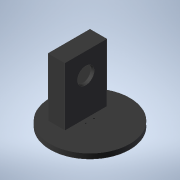
# Autodesk Inventor part: NBase top
Saved by Autodesk Inventor 2022 (Build 260153000, 153)
## iProperties
Created: 2022-02-11
Part Number: NBase top
Material: Generic
Document SubType Name: Modeling
Designer: Alexa
Density: 1 g/cm^3
Appearance: Default
Author: Alexa
Autodesk Inventor part; units mm, degrees
ref_plane "YZ Plane" through (0, 0, 0) normal (1, 0, 0) x (0, 1, 0)
ref_plane "XZ Plane" through (0, 0, 0) normal (0, 1, 0) x (-1, 0, 0)
ref_plane "XY Plane" through (0, 0, 0) normal (0, 0, 1) x (1, 0, 0)
sketch "Sketch1" plane through (0, 0, 0) normal (0, 1, 0) x (-1, 0, 0)
  circle A0 centre (0, 0) radius 47.5
  dimension "d0" = 95
  constraints: 1 centre point, 1 coincident
  measures "d0" diameter of A0
extrude "Extrusion1" add sketch "Sketch1" along normal blind 6
sketch "Sketch2" plane through (0, 6, 0) normal (0, 1, 0) x (1, 0, 0)
  circle A0 centre (0, 0) radius 10
  circle A1 centre (0, 5) radius 1
  circle A2 centre (0, -5) radius 1
  dimension "d3" = 20
  dimension "d4" = 2
  dimension "d5" = 2
  constraints: 3 centre point, 1 coincident
  measures "d3" diameter of A0
  measures "d4" diameter of A1
  measures "d5" diameter of A2
extrude "Extrusion2" cut sketch "Sketch2" against normal blind 23.4625 contours A1 | A2
sketch "Sketch3" plane through (0, 0, 0) normal (0, -1, 0) x (1, 0, 0)
  circle A0 centre (0, 0) radius 10
  constraints: 1 centre point, 1 coincident
sketch "Sketch4" plane through (0, 6, 0) normal (0, 1, 0) x (1, 0, 0)
  line L0 (0, 0) -> (-10, 0)
  line L1 (-10, 0) -> (-10, 25)
  line L2 (-10, 25) -> (0, 25)
  line L3 (0, 25) -> (0, 0)
  line L4 (0, 0) -> (-5, 0)
  line L5 (-5, 0) -> (-5, 25)
  line L6 (-5, 25) -> (0, 25)
  line L7 (0, 25) -> (0, 0)
  line L8 (-5, 25) -> (-20, 25)
  line L9 (-20, 25) -> (-20, -25)
  line L10 (-20, -25) -> (-5, -25)
  line L11 (-5, -25) -> (-5, 25)
  line L12 (-5, 25) -> (-25, 25)
  line L13 (-25, 25) -> (-25, -25)
  line L14 (-25, -25) -> (-5, -25)
  line L15 (-5, -25) -> (-5, 25)
  dimension "d9" = 10
  dimension "d10" = 25
  dimension "d11" = 15
  dimension "d12" = 50
  dimension "d13" = 20
  constraints: 32 end point, 8 parallel, 4 horizontal, 4 perpendicular, 1 midpoint
  measures "d9" distance of L1.end L2.end
  measures "d10" distance of L0.end L1.end
  measures "d11" distance of L10.end L9.end
  measures "d12" distance of L9.end L8.end
  measures "d13" distance of L14.end L13.end
extrude "Extrusion3" add sketch "Sketch4" along normal blind 70 contours L11 L10 L9 L8 L1 L0 | L0 L1 L2 L5 | L14 L13 L12 L9
sketch "Sketch5" plane through (-25, 6, -25) normal (-1, 0, 0) x (0, 0, 1)
  line L0 (0, 0) -> (0, 70) projected
  line L1 (50, 0) -> (50, 70) projected
  line L2 (0, 70) -> (50, 70)
  line L3 (50, 70) -> (50, 0)
  line L4 (50, 0) -> (0, 0)
  line L5 (0, 0) -> (0, 70)
  line L6 (50, 70) -> (0, 70) projected
  line L7 (72.5, 0) -> (-22.5, 0) projected
  line L8 (0, 70) -> (25, 70)
  line L9 (25, 70) -> (25, 0)
  line L10 (25, 0) -> (0, 0)
  line L11 (0, 0) -> (0, 70)
  line L12 (25, 35) -> (15, 35)
  line L13 (15, 35) -> (15, 15)
  line L14 (15, 15) -> (25, 15)
  line L15 (25, 15) -> (25, 35)
  line L16 (15, 35) -> (25, 35)
  line L17 (25, 35) -> (25, 55)
  line L18 (25, 55) -> (15, 55)
  line L19 (15, 55) -> (15, 35)
  line L20 (15, 15) -> (35, 15)
  line L21 (35, 15) -> (35, 55)
  line L22 (35, 55) -> (15, 55)
  line L23 (15, 55) -> (15, 15)
  line L24 (15, 15) -> (35, 15)
  line L25 (35, 15) -> (35, 55.5)
  line L26 (35, 55.5) -> (15, 55.5)
  line L27 (15, 55.5) -> (15, 15)
  point P0 (25, -6)
  dimension "d16" = 10
  dimension "d17" = 20
  dimension "d18" = 20
  dimension "d19" = 20
  dimension "d20" = 40.5
  constraints: 48 end point, 12 parallel, 6 horizontal, 6 perpendicular, 3 point on line, 2 midpoint
  measures "d16" distance of L14.end L13.end
  measures "d17" distance of L13.end L12.end
  measures "d18" distance of L17.end L16.end
  measures "d19" distance of L22.end L21.end
  measures "d20" distance of L25.end L24.end
extrude "Extrusion4" cut sketch "Sketch5" against normal blind 16 contours L14 L13 L12 L9 | L9 L22 L21 L20 | L26 L25 L22 L9 | L9 L18 L27 L26 | L12 L19 L18 L9
sketch "Sketch6" plane through (-25, 6, -25) normal (-1, 0, 0) x (0, 0, 1)
  line L0 (35, 15) -> (15, 15) projected
  line L1 (15, 15) -> (35, 15)
  line L2 (35, 15) -> (35, 9)
  line L3 (35, 9) -> (15, 9)
  line L4 (15, 9) -> (15, 15)
  line L5 (15, 55.5) -> (35, 55.5) projected
  line L6 (15, 55.5) -> (35, 55.5)
  line L7 (35, 55.5) -> (35, 61.5)
  line L8 (35, 61.5) -> (15, 61.5)
  line L9 (15, 61.5) -> (15, 55.5)
  point P0 (25, -6)
  dimension "d23" = 6
  dimension "d24" = 6
  constraints: 16 end point, 4 parallel, 2 horizontal, 2 perpendicular, 1 point on line
  measures "d23" distance of L1.end L2.end
  measures "d24" distance of L7.end L6.end
extrude "Extrusion5" cut sketch "Sketch6" against normal blind 6
sketch "Sketch7" plane through (-19, 6, -25) normal (-1, 0, 0) x (0, 0, 1)
  line L0 (35, 9) -> (15, 9) projected
  line L1 (35, 61.5) -> (35, 9) projected
  line L2 (15, 9) -> (35, 9)
  line L3 (35, 9) -> (35, 11.6)
  line L4 (35, 11.6) -> (15, 11.6)
  line L5 (15, 11.6) -> (15, 9)
  line L6 (15, 55.5) -> (15, 61.5) projected
  line L7 (35, 61.5) -> (35, 55.5) projected
  line L8 (15, 61.5) -> (35, 61.5)
  line L9 (35, 61.5) -> (35, 58.5)
  line L10 (35, 58.5) -> (15, 58.5)
  line L11 (15, 58.5) -> (15, 61.5)
  line L12 (15, 9) -> (15, 61.5) projected
  line L13 (15, 9) -> (35, 9)
  line L14 (35, 9) -> (35, 12)
  line L15 (35, 12) -> (15, 12)
  line L16 (15, 12) -> (15, 9)
  line L17 (35, 15) -> (15, 15) projected
  line L18 (25, 15) -> (20, 15)
  line L19 (20, 15) -> (20, 12)
  line L20 (20, 12) -> (25, 12)
  line L21 (25, 12) -> (25, 15)
  line L22 (25, 15) -> (30, 15)
  line L23 (30, 15) -> (30, 12)
  line L24 (30, 12) -> (25, 12)
  line L25 (25, 12) -> (25, 15)
  line L26 (15, 61.5) -> (35, 61.5) projected
  line L27 (25, 58.5) -> (20, 58.5)
  line L28 (20, 58.5) -> (20, 61.5)
  line L29 (20, 61.5) -> (25, 61.5)
  line L30 (25, 61.5) -> (25, 58.5)
  line L31 (25, 58.5) -> (30, 58.5)
  line L32 (30, 58.5) -> (30, 61.5)
  line L33 (30, 61.5) -> (25, 61.5)
  line L34 (25, 61.5) -> (25, 58.5)
  circle A0 centre (20, 12) radius 1.35
  circle A1 centre (30, 12) radius 1.35
  circle A2 centre (20, 58.5) radius 1.35
  circle A3 centre (30, 58.5) radius 1.35
  point P0 (25, -6)
  dimension "d27" = 2.6
  dimension "d28" = 3
  dimension "d29" = 3
  dimension "d30" = 5
  dimension "d31" = 5
  dimension "d32" = 2.7
  dimension "d33" = 2.7
  dimension "d34" = 2.7
  dimension "d35" = 2.7
  constraints: 56 end point, 14 parallel, 8 point on line, 7 horizontal, 7 perpendicular, 4 centre point, 4 coincident, 3 midpoint
  measures "d27" distance of L3.end L2.end
  measures "d28" distance of L8.end L9.end
  measures "d29" distance of L14.end L13.end
  measures "d30" distance of L20.end L19.end
  measures "d31" distance of L23.end L24.end
  measures "d32" diameter of A0
  measures "d33" diameter of A1
  measures "d34" diameter of A2
  measures "d35" diameter of A3
extrude "Extrusion6" cut sketch "Sketch7" against normal blind 10 contours A1 L4 | L4 A1 L15 | A0 L15 L4 | L4 A0 | L15 L23 A1 | A0 L19 L15 | L15 A1 L23 | L15 L19 A0 | A3 L10 | L10 L32 A3 | A2 L28 L10 | L10 A2 | L10 A3 L32 | L28 A2 L10
thread "Thread1" size "M3x0.5" class "6H" standard "ANSI Metric M Profile" full length
thread "Thread2" size "M3x0.5" class "6H" standard "ANSI Metric M Profile" full length
thread "Thread3" size "M3x0.5" class "6H" standard "ANSI Metric M Profile" full length
thread "Thread4" size "M3x0.5" class "6H" standard "ANSI Metric M Profile" full length
sketch "Sketch8" plane through (-9, 6, -25) normal (-1, 0, 0) x (0, 0, 1)
  line L0 (15, 9) -> (15, 61.5) projected
  line L1 (35, 55.5) -> (35, 15) projected
  line L2 (15, 61.5) -> (35, 61.5)
  line L3 (35, 61.5) -> (35, 44.5)
  line L4 (35, 44.5) -> (15, 44.5)
  line L5 (15, 44.5) -> (15, 61.5)
  circle A0 centre (25, 44.5) radius 10
  point P0 (25, -6)
  dimension "d46" = 17
  dimension "d47" = 20
  constraints: 8 end point, 2 parallel, 1 centre point, 1 horizontal, 1 midpoint, 1 perpendicular, 1 point on line
  measures "d46" distance of L2.end L3.end
  measures "d47" diameter of A0
extrude "Extrusion7" cut sketch "Sketch8" against normal blind 15.4 contours A0 L4 | L4 A0
body "Solid1"
